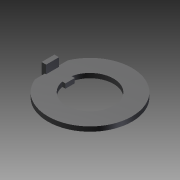
# Autodesk Inventor part: AT518
Saved by Autodesk Inventor 2011 SP1 (Build 150282100, 282)
## iProperties
Created: 2016-09-01
Part Number: AT518
Catalog Web Link: www.cadenas.de
Description: AT518 - Locking Ring-
Vendor: NKKSWITCHES
Document SubType Name: Modeling
Designer: psAdmin
Manufacturer: NKKSWITCHES
Mass: 0.181686 g
Surface Area: 4.61001 cm^2
Volume: 0.181686 cm^3
Density: 1 g/cm^3
Category: PARTsolutions
Company: NKKSWITCHES
Title: AT518
Author: Cadenas PARTsolutions
PSOL_IDENT_0: {$CADENAS_DATA\23d-libs\nkkswitches\rotary\hs_12_amp\parts\at518.prj},166 {VTYP=3D},{NB=AT518},{LINA=
PSOL_IDENT_1: AT518},{NN=AT518 - Locking Ring},{DATE=22.09.2015 06:04:15},{GEOMDATE=27.03.2009 08:30:00},{VERSION=
PSOL_IDENT_2: },{LINEID=10},{LINESUBID=-1},{WBVAR=}  {NB=AT518},{LINA=AT518},{KT=DUMMY},{PN=AT518}
NN: AT518 - Locking Ring
NB: AT518
NBSYN: $PN.
LINA: AT518
PN: AT518
SUPPLIER: NKKSWITCHES
ARTICLENO: AT518
BOMINFO: AT518
CREATOR: CADENAS GmbH
Autodesk Inventor part; units mm, degrees
sketch "Sketch_1" plane through (0, 0, 0) normal (0, 1, 0) x (-1, 0, 0)
  line L0 (8.382, -3.558) -> (8.382, 3.558)
  arc A0 (8.382, 3.558) -> (8.382, -3.558) centre (0, 0) ccw
  arc A1 (5.0033, 1.016) -> (5.0033, -1.016) centre (0, 0) ccw
  line L1 (5.0033, -1.016) -> (4.3053, -1.016)
  line L2 (4.3053, -1.016) -> (4.3053, 1.016)
  line L3 (4.3053, 1.016) -> (5.0033, 1.016)
  constraints: 8 end point, 4 point on circle, 2 centre point
extrude "Extrusion1" add sketch "Sketch_1" along normal mid plane 0.9906
sketch "Sketch_2" plane through (0, 0, 0) normal (0, 0, 1) x (1, 0, 0)
  arc A0 (-9.1059, 0.2667) -> (-8.3439, -0.4953) centre (-8.3439, 0.2667) ccw
  line L0 (-8.3439, -0.4953) -> (-8.1153, -0.4953)
  line L1 (-8.1153, -0.4953) -> (-8.1153, 2.2987)
  line L2 (-8.1153, 2.2987) -> (-9.1059, 2.2987)
  line L3 (-9.1059, 2.2987) -> (-9.1059, 0.2667)
  constraints: 8 end point, 2 point on circle, 1 centre point
extrude "Extrusion2" add sketch "Sketch_2" along normal mid plane 2.794
ref_plane "1_XY" through (0, 0, 0) normal (0, 1, 0) x (1, 0, 0)
ref_plane "1_YZ" through (0, 0, 0) normal (1, 0, 0) x (0, 0, -1)
ref_plane "1_ZX" through (0, 0, 0) normal (0, 0, -1) x (0, 1, 0)
body "Solid1"
